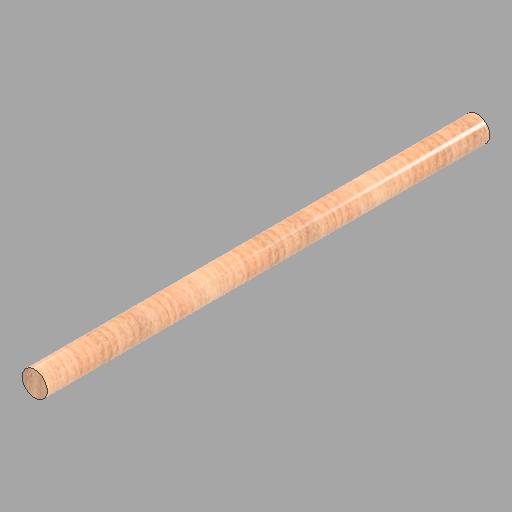
# Autodesk Inventor part: PIPE LONG
Saved by Autodesk Inventor 2025.2 (Build 292293000, 293)
## iProperties
Created: 2025-01-29
Part Number: PIPE LONG
Material: Wood (Birch)
Document SubType Name: Modeling
Designer: Anna
Density: 0.55 g/cm^3
Appearance: Birch - Natural Polished
Mass: 422.068 g
Surface Area: 828.467 cm^2
Volume: 767.396 cm^3
Author: Anna
Autodesk Inventor part; units mm, degrees
ref_plane "YZ Plane" through (0, 0, 0) normal (1, 0, 0) x (0, 1, 0)
sketch "Sketch1" plane through (0, 0, 0) normal (0, 0, 1) x (1, 0, 0)
  circle A0 centre (0, 141) radius 19.05
  point P0 (0, 0)
  dimension "d3" = 38.1
  constraints: 1 centre point
  measures "d3" diameter of A0
ref_plane "Work Plane1" through (-139.7, -1066.8, 927.1) normal (0, 0, -1) x (0, 1, 0)
ref_plane "Work Plane2" through (-139.7, -1753.9498, 673.1) normal (0, 0, -1) x (0, 1, 0)
extrude "Extrusion1" add sketch "Sketch1" along normal up to surface (673.1 mm away)
body "Solid1"
